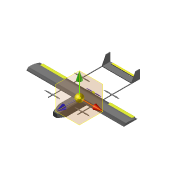
# Autodesk Inventor part: tesagain
Saved by Autodesk Inventor 2020 (Build 240168000, 168)
## iProperties
Part Number: tesagain
Material: Generic
Document SubType Name: Modeling
Designer: alifhabib
Appearance: Default
Mass: 27084.8 g
Surface Area: 16926.9 cm^2
Volume: 27084.8 cm^3
Density: 1 g/cm^3
Author: alifhabib
Autodesk Inventor part; units mm, degrees
sketch "Sketch1" plane through (0, 0, 0) normal (1, 0, 0) x (0, 1, 0)
  line L0 (-75, 187.5) -> (-75, -287.5)
  line L1 (75, -287.5) -> (75, 187.5)
  line L2 (75, 187.5) -> (-75, 187.5)
  line L3 (75, -287.5) -> (-75, -287.5)
  line L4 (75, -287.5) -> (75, -287.5)
  point P0 (0, 0)
  dimension "d5" = 150
  dimension "d15" = 0
  constraints: 10 end point, 2 perpendicular, 1 parallel, 1 vertical
  measures "d5" distance of L1.end L0.start
  measures "d15" distance of L1.start L4.end
extrude "Extrusion1" add sketch "Sketch1" along normal mid plane 150
ref_plane "Work Plane1" through (-75, -75, 337.5) normal (0, 0, 1) x (1, 0, 0)
sketch "Sketch2" plane through (-75, -75, 337.5) normal (0, 0, 1) x (1, 0, 0)
  line L0 (35, 115) -> (115, 115)
  line L1 (115, 115) -> (115, 35)
  line L2 (115, 35) -> (35, 35)
  line L3 (35, 35) -> (35, 115)
  line L4 (35, 115) -> (115, 35) construction
  line L5 (115, 115) -> (35, 35) construction
  point P0 (75, 75)
  dimension "d9" = 80
  dimension "d10" = 80
  constraints: 12 end point, 2 midpoint, 2 parallel, 1 horizontal, 1 perpendicular
  measures "d9" distance of L1.end L2.end
  measures "d10" distance of L0.end L1.end
loft "Loft1" add profiles "Sketch2" section 2 edges at (0, -75, 187.5) (75, 0, 187.5) (0, 75, 187.5) (-75, 0, 187.5)
ref_plane "Work Plane2" through (75, 75, -337.5) normal (0, 0, -1) x (-1, 0, 0)
sketch "Sketch3" plane through (75, 75, -337.5) normal (0, 0, -1) x (-1, 0, 0)
  line L0 (40, -40) -> (110, -40)
  line L1 (110, -40) -> (110, -110)
  line L2 (110, -110) -> (40, -110)
  line L3 (40, -110) -> (40, -40)
  line L4 (40, -40) -> (110, -110) construction
  line L5 (110, -40) -> (40, -110) construction
  point P0 (75, -75)
  dimension "d17" = 70
  dimension "d18" = 70
  constraints: 12 end point, 2 midpoint, 2 parallel, 1 horizontal, 1 perpendicular
  measures "d17" distance of L1.end L2.end
  measures "d18" distance of L0.end L1.end
loft "Loft2" add profiles "Sketch3" section 2 edges at (0, 75, -287.5) (75, 0, -287.5) (0, -75, -287.5) (-75, 0, -287.5)
fillet "Fillet1" radius 20 20 edges at (75, 75, -50) (55, 55, -312.5) (-55, 55, -312.5) (-75, 75, -50) (57.5, 57.5, 262.5) (-57.5, 57.5, 262.5) (57.5, -57.5, 262.5) (75, -75, -50) (55, -55, -312.5) (-55, -55, -312.5) (-75, -75, -50) (0, 40, 337.5) (0, -40, 337.5) (-57.5, -57.5, 262.5) (40, 0, 337.5) (-40, 0, 337.5) (0, 35, -337.5) (35, 0, -337.5) (0, -35, -337.5) (-35, 0, -337.5)
sketch "Sketch4" plane through (0, 0, 0) normal (1, 0, 0) x (0, 1, 0)
  line L0 (41.0049, -329.9939) -> (74.5995, -288.0006) projected
  line L1 (74.5995, -38.0006) -> (74.5995, -288.0006)
  arc A0 (114.5995, -75.8397) -> (74.5995, -38.0006) centre (7.1799, -149.332) ccw
  arc A1 (74.5995, -288.0006) -> (114.5995, -75.8397) centre (-339.3185, -100.1109) ccw
  point P0 (0, 0)
  constraints: 4 point on circle, 2 centre point, 2 end point
extrude "Extrusion2" add sketch "Sketch4" along normal mid plane 1800
sketch "Sketch5" plane through (-55, 75, 187.5) normal (0, 1, 0) x (1, 0, 0)
  line L0 (110, 475) -> (0, 475) projected
  line L1 (55, 475) -> (322.5, 475)
  line L2 (322.5, 475) -> (332.5, 475)
  line L3 (332.5, 475) -> (332.5, 1145)
  line L4 (332.5, 1145) -> (322.5, 1145)
  line L5 (322.5, 1145) -> (322.5, 475)
  line L6 (322.5, 1145) -> (-212.5, 1145)
  line L7 (-212.5, 1145) -> (-212.5, 995)
  line L8 (-212.5, 995) -> (322.5, 995)
  line L9 (322.5, 995) -> (322.5, 1145)
  line L10 (-212.5, 1145) -> (-222.5, 1145)
  line L11 (-222.5, 1145) -> (-222.5, 475)
  line L12 (-222.5, 475) -> (-212.5, 475)
  line L13 (-212.5, 475) -> (-212.5, 1145)
  point P0 (55, 187.5)
  dimension "d28" = 267.5
  dimension "d29" = 10
  dimension "d30" = 670
  dimension "d31" = 535
  dimension "d32" = 150
  dimension "d33" = 10
  constraints: 26 end point, 6 parallel, 3 horizontal, 3 perpendicular, 1 collinear, 1 midpoint
  measures "d28" distance of L1.start L1.end
  measures "d29" distance of L4.end L3.end
  measures "d30" distance of L3.end L2.end
  measures "d31" distance of L8.end L7.end
  measures "d32" distance of L7.end L6.end
  measures "d33" distance of L12.end L11.end
extrude "Extrusion3" add sketch "Sketch5" against normal blind 10
sketch "Sketch6" plane through (277.5, 75, -287.5) normal (1, 0, 0) x (0, 0, -1)
  line L0 (0, 0) -> (670, 0) projected
  line L1 (670, 0) -> (670, 150)
  line L2 (670, 150) -> (595, 150)
  line L3 (670, 0) -> (520, 0)
  line L4 (520, 0) -> (595, 150)
  point P0 (-287.5, -75)
  dimension "d36" = 150
  dimension "d37" = 75
  dimension "d38" = 150
  constraints: 8 end point, 1 perpendicular, 1 point on line, 1 vertical
  measures "d36" distance of L0.end L1.end
  measures "d37" distance of L1.end L2.end
  measures "d38" distance of L0.end L3.end
extrude "Extrusion4" add sketch "Sketch6" against normal blind 10
mirror "Mirror1" about plane through (0, 0, 0) normal (1, 0, 0) of "Extrusion4"
sketch "Sketch7" plane through (58.9822, 74.5995, -38.0006) normal (0, -1, 0) x (1, 0, 0)
  line L0 (208.5178, -249.4994) -> (218.5178, -249.4994) projected
  line L1 (208.5178, -249.4994) -> (218.5178, -249.4994)
  line L2 (218.5178, -249.4994) -> (218.5178, 225.5006)
  line L3 (218.5178, 225.5006) -> (208.5178, 225.5006)
  line L4 (208.5178, 225.5006) -> (208.5178, -249.4994)
  line L5 (-326.4822, -249.4994) -> (-336.4822, -249.4994) projected
  line L6 (-336.4822, -249.4994) -> (-326.4822, -249.4994)
  line L7 (-326.4822, -249.4994) -> (-326.4822, 225.5006)
  line L8 (-326.4822, 225.5006) -> (-336.4822, 225.5006)
  line L9 (-336.4822, 225.5006) -> (-336.4822, -249.4994)
  point P0 (-58.9822, 38.0006)
  dimension "d41" = 10
  dimension "d42" = 475
  dimension "d43" = 10
  dimension "d44" = 475
  constraints: 16 end point, 4 parallel, 2 horizontal, 2 perpendicular
  measures "d41" distance of L3.end L2.end
  measures "d42" distance of L2.end L1.end
  measures "d43" distance of L8.end L7.end
  measures "d44" distance of L7.end L6.end
extrude "Extrusion5" add sketch "Sketch7" along normal blind 10
sketch "Sketch8" plane through (58.9822, 74.5995, -38.0006) normal (0, 1, 0) x (1, 0, 0)
  line L0 (-336.4822, 250) -> (-336.4822, 0) projected
  line L1 (-336.4822, 0) -> (-336.4822, -150)
  line L2 (-336.4822, -225.5006) -> (-336.4822, 0) projected
  line L3 (-336.4822, 769.4994) -> (-336.4822, 249.4994) projected
  line L4 (-336.4822, 249.4994) -> (-336.4822, 399.4994)
  line L5 (-336.4822, 399.4994) -> (-326.4822, 399.4994)
  line L6 (-326.4822, 249.4994) -> (-326.4822, 769.4994) projected
  circle A0 centre (-331.4822, 399.4994) radius 20
  line L7 (-336.4822, 399.4994) -> (-476.4822, 399.4994)
  arc A1 (-476.4822, 399.4994) -> (-336.4822, 399.4994) centre (-406.4822, 711.578) ccw
  arc A2 (-336.4822, 399.4994) -> (-476.4822, 399.4994) centre (-406.4822, 250.3822) ccw
  line L8 (-331.4822, 399.4994) -> (-331.4822, 405.4154)
  arc A3 (-326.4822, 399.4994) -> (-186.4822, 399.4994) centre (-256.4822, 711.578) ccw
  arc A4 (-186.4822, 399.4994) -> (-326.4822, 399.4994) centre (-256.4822, 250.3822) ccw
  line L9 (-336.4822, -300) -> (-336.4822, -150)
  line L10 (-336.4822, -150) -> (-326.4822, -150)
  circle A5 centre (-331.4822, -150) radius 20
  line L11 (-336.4822, -150) -> (-476.4822, -150)
  arc A6 (-476.4822, -150) -> (-336.4822, -150) centre (-406.4822, 162.0785) ccw
  arc A7 (-336.4822, -150) -> (-476.4822, -150) centre (-406.4822, -299.1172) ccw
  line L12 (-331.4822, -150) -> (-331.4822, -144.084)
  arc A8 (-326.4822, -150) -> (-186.4822, -150) centre (-256.4822, 162.0785) ccw
  arc A9 (-186.4822, -150) -> (-326.4822, -150) centre (-256.4822, -299.1172) ccw
  line L13 (208.2747, 249.4994) -> (208.2747, 399.4994)
  line L14 (208.2747, 399.4994) -> (218.2747, 399.4994)
  circle A10 centre (213.2747, 399.4994) radius 20
  line L15 (208.2747, 399.4994) -> (68.2747, 399.4994)
  arc A11 (68.2747, 399.4994) -> (208.2747, 399.4994) centre (138.2747, 711.578) ccw
  arc A12 (208.2747, 399.4994) -> (68.2747, 399.4994) centre (138.2747, 250.3822) ccw
  line L16 (213.2747, 399.4994) -> (213.2747, 405.4154)
  arc A13 (218.2747, 399.4994) -> (358.2747, 399.4994) centre (288.2747, 711.578) ccw
  arc A14 (358.2747, 399.4994) -> (218.2747, 399.4994) centre (288.2747, 250.3822) ccw
  arc A15 (218.2747, -150) -> (358.2747, -150) centre (288.2747, 162.0785) ccw
  arc A16 (358.2747, -150) -> (218.2747, -150) centre (288.2747, -299.1172) ccw
  line L17 (208.2747, -150) -> (218.2747, -150)
  line L18 (213.2747, -150) -> (213.2747, -144.084)
  circle A17 centre (213.2747, -150) radius 20
  line L19 (208.2747, -150) -> (68.2747, -150)
  arc A18 (68.2747, -150) -> (208.2747, -150) centre (138.2747, 162.0785) ccw
  arc A19 (208.2747, -150) -> (68.2747, -150) centre (138.2747, -299.1172) ccw
  point P0 (-58.9822, -38.0006)
  dimension "d47" = 150
  dimension "d53" = 150
  dimension "d54" = 40
  dimension "d55" = 140
  dimension "d56" = 150
  dimension "d57" = 40
  dimension "d58" = 140
  dimension "d59" = 150
  dimension "d60" = 40
  dimension "d61" = 140
  dimension "d62" = 40
  dimension "d63" = 140
  constraints: 32 end point, 32 point on circle, 20 centre point, 12 symmetric about line, 8 horizontal, 4 midpoint, 4 vertical, 3 point on line, 8 other
  measures "d47" distance of L0.end L1.end
  measures "d53" distance of L3.end L4.end
  measures "d54" diameter of A0
  measures "d55" distance of L4.end L7.end
  measures "d56" distance of L9.start L9.end
  measures "d57" diameter of A5
  measures "d58" distance of L9.end L11.end
  measures "d59" distance of L13.start L13.end
  measures "d60" diameter of A10
  measures "d61" distance of L13.end L15.end
  measures "d62" diameter of A17
  measures "d63" distance of L19.start L19.end
extrude "Extrusion6" add sketch "Sketch8" along normal blind 4
ref_plane "Work Plane3" through (25.3875, -25.3875, -337.5) normal (0, 0, -1) x (-1, 0, 0)
sketch "Sketch9" plane through (25.3875, -25.3875, -337.5) normal (0, 0, -1) x (-1, 0, 0)
  circle A0 centre (25.3875, 25.3875) radius 25
  dimension "d67" = 50
  constraints: 1 centre point, 1 coincident
  measures "d67" diameter of A0
extrude "Extrusion7" add sketch "Sketch9" along normal blind 40
sketch "Sketch10" plane through (0, 0, -377.5) normal (0, 0, -1) x (-1, 0, 0)
  circle A0 centre (0, 0) radius 15
  line L0 (-15, 0) -> (-135, 0)
  arc A1 (-15, 0) -> (-135, 0) centre (-75, -279.5962) ccw
  arc A2 (-135, 0) -> (-15, 0) centre (-75, 380.0107) ccw
  line L1 (0, 0) -> (0, 7.7101)
  line L2 (15, 0) -> (135, 0)
  arc A3 (135, 0) -> (15, 0) centre (75, -279.5962) ccw
  arc A4 (15, 0) -> (135, 0) centre (75, 380.0107) ccw
  dimension "d70" = 30
  dimension "d71" = 120
  constraints: 8 point on circle, 6 end point, 4 centre point, 4 symmetric about line, 1 coincident, 1 horizontal, 1 horizontal alignment, 1 vertical, 4 other
  measures "d71" distance of L0.start L0.end
extrude "Extrusion8" add sketch "Sketch10" along normal blind 10 contours A0 | A2 L0 | L0 A1 | A3 L2
sketch "Sketch11" plane through (-55, 75, 187.5) normal (0, 1, 0) x (1, 0, 0)
  line L0 (-212.5, 1145) -> (-212.5, 995) projected
  line L1 (-212.5, 1145) -> (-162.5, 1145)
  line L2 (-222.5, 1145) -> (332.5, 1145) projected
  line L3 (322.5, 1145) -> (272.5, 1145)
  line L4 (-162.5, 1145) -> (272.5, 1145)
  line L5 (272.5, 1145) -> (272.5, 1105)
  line L6 (272.5, 1105) -> (-162.5, 1105)
  line L7 (-162.5, 1105) -> (-162.5, 1145)
  point P0 (55, 187.5)
  dimension "d74" = 50
  dimension "d75" = 50
  dimension "d76" = 40
  constraints: 12 end point, 2 parallel, 2 point on line, 1 horizontal, 1 perpendicular
  measures "d74" distance of L0.start L1.end
  measures "d75" distance of L3.start L3.end
  measures "d76" distance of L4.end L5.end
extrude "Extrusion9" cut sketch "Sketch11" against normal blind 10
sketch "Sketch12" plane through (-55, 75, 187.5) normal (0, 1, 0) x (1, 0, 0)
  line L0 (322.5, 1145) -> (272.5, 1145)
  line L1 (-162.5, 1150.1057) -> (272.5, 1150.1057)
  line L2 (272.5, 1150.1057) -> (272.5, 1110.1057)
  line L3 (272.5, 1110.1057) -> (-162.5, 1110.1057)
  line L4 (-162.5, 1110.1057) -> (-162.5, 1150.1057)
  point P0 (55, 187.5)
  point P1 (332.5, 1145)
  dimension "d79" = 50
  dimension "d80" = 40
  constraints: 10 end point, 2 parallel, 1 horizontal, 1 perpendicular
  measures "d79" distance of L0.start L0.end
  measures "d80" distance of L1.end L2.end
extrude "Extrusion10" add sketch "Sketch12" against normal mid plane 10
sketch "Sketch13" plane through (217.5, 75, -922.6057) normal (1, 0, 0) x (0, 0, -1)
  line L0 (40, 5) -> (0, 5) projected
  line L1 (40, -5) -> (40, 0)
  line L2 (34.8943, -5) -> (40, -5) projected
  line L3 (40, 0) -> (34.8943, -5)
  line L4 (34.8943, -5) -> (40, -7.8447)
  line L5 (40, -7.8447) -> (44.3121, -2.2073)
  line L6 (40, 0) -> (34.8943, 5)
  line L7 (34.8943, 150) -> (34.8943, 0) projected
  line L8 (39.5176, 7.5389) -> (43.2545, 7.5389)
  line L9 (39.5176, 7.5389) -> (34.8943, 5)
  line L10 (40, 0) -> (44.3121, -2.2073)
  line L11 (43.2545, 7.6661) -> (40, 0)
  point P0 (-922.6057, -75)
  point P1 (43.2005, 7.5389)
  constraints: 18 end point, 3 point on line, 1 horizontal
extrude "Extrusion11" cut sketch "Sketch13" against normal blind 1000
sketch "Sketch14" plane through (900, 74.5995, -288.0006) normal (0, -1, 0) x (1, 0, 0)
  line L0 (0, 0) -> (0, 212.1609) projected
  line L1 (0, 0) -> (-50, 0)
  line L2 (-622.5, 0) -> (0, 0) projected
  line L3 (-50, 0) -> (-500, 0)
  line L4 (-500, 0) -> (-500, 60)
  line L5 (-500, 60) -> (-50, 60)
  line L6 (-50, 60) -> (-50, 0)
  point P0 (-900, 288.0006)
  point P1 (-500, 0)
  dimension "d87" = 50
  dimension "d88" = 450
  dimension "d89" = 60
  constraints: 10 end point, 2 parallel, 1 horizontal, 1 perpendicular, 1 point on line
  measures "d87" distance of L0.start L1.end
  measures "d88" distance of L4.end L5.end
  measures "d89" distance of L3.end L4.end
extrude "Extrusion12" cut sketch "Sketch14" against normal blind 190
mirror "Mirror2" about plane through (0, 0, 0) normal (1, 0, 0) of "Extrusion12"
sketch "Sketch15" plane through (900, 74.5995, -288.0006) normal (0, -1, 0) x (1, 0, 0)
  line L0 (-50, 60) -> (-50, 0) projected
  line L1 (-50, 60) -> (-50, 50)
  line L2 (-50, 50) -> (-500, 50)
  line L3 (-500, 50) -> (-500, -10)
  line L4 (-500, -10) -> (-50, -10)
  line L5 (-50, -10) -> (-50, 50)
  point P0 (-900, 288.0006)
  dimension "d92" = 10
  dimension "d93" = 450
  dimension "d94" = 60
  constraints: 10 end point, 2 parallel, 1 horizontal, 1 perpendicular, 1 point on line
  measures "d92" distance of L0.start L1.end
  measures "d93" distance of L4.end L3.end
  measures "d94" distance of L3.end L2.end
extrude "Extrusion13" add sketch "Sketch15" against normal blind 10
sketch "Sketch16" plane through (850, 74.5995, -288.0006) normal (1, 0, 0) x (0, 0, -1)
  line L0 (10, 10) -> (-23.8038, 10) projected
  line L1 (10, 10) -> (0, 10)
  line L2 (0, 10) -> (10, 5)
  line L3 (10, 0) -> (10, 10) projected
  line L4 (-250, 0) -> (0, 0) projected
  line L5 (10, 5) -> (0, 0)
  line L6 (0, 0) -> (11.584, -3.5959)
  line L7 (11.584, -3.5959) -> (15.1909, 5)
  line L8 (15.1909, 5) -> (10, 5)
  line L9 (14.663, 9.6441) -> (10, 5)
  line L10 (0, 10) -> (13.1045, 11.209)
  line L11 (13.1045, 11.209) -> (14.663, 9.6441)
  point P0 (-288.0006, -74.5995)
  dimension "d97" = 10
  constraints: 18 end point, 1 midpoint, 1 parallel, 1 perpendicular, 1 point on line
  measures "d97" distance of L0.start L1.end
extrude "Extrusion14" cut sketch "Sketch16" against normal blind 1000
mirror "Mirror3" about plane through (0, 0, 0) normal (1, 0, 0) of "Extrusion14", "Extrusion13"
body "Solid1"
